BUCK_MODULE (Autodesk Fusion 360 design; units mm, degrees)
Autodesk Fusion 360 part; units mm, degrees
note: some values were not read from the file. Set by a fixed rule: which sketch regions a step uses.
sketch "Esquisse1" plane through (0, 0, 0) normal (0, 0, 1) x (1, 0, 0)
  line L0 (38, -53) -> (-38, -53)
  line L1 (-38, -53) -> (-38, 53)
  line L2 (-38, 53) -> (38, 53)
  line L3 (38, 53) -> (38, -53)
  line L4 (38, -53) -> (-38, 53) construction
  line L5 (-38, -53) -> (38, 53) construction
  dimension "d1" = 76
  dimension "d2" = 106
  constraint horizontal L0
  constraint perpendicular L0 L1
  constraint parallel L0 L2
  constraint parallel L1 L3
  constraint coincident L4 origin
  constraint coincident L5 origin
  measures "d1" distance of L1.end L2.end
  measures "d2" distance of L0.end L1.end
extrude "Extrusion1" add sketch "Esquisse1" along normal blind 40
sketch "Esquisse2" plane through (0, 0, 0) normal (0, 0, -1) x (1, 0, 0)
  line L0 (-38, -53) -> (38, -53)
  line L1 (38, -53) -> (38, 53)
  line L2 (38, 53) -> (-38, 53)
  line L3 (-38, 53) -> (-38, -53)
  line L4 (34.75, -38) -> (-34.75, -38)
  line L5 (-34.75, -38) -> (-34.75, 49)
  line L6 (-34.75, 49) -> (34.75, 49)
  line L7 (34.75, 49) -> (34.75, -38)
  line L8 (34.75, -38) -> (-34.75, 49) construction
  line L9 (-34.75, -38) -> (34.75, 49) construction
  line L10 (-34.75, -38) -> (34.75, -38)
  line L11 (34.75, -38) -> (34.75, -49)
  line L12 (34.75, -49) -> (-34.75, -49)
  line L13 (-34.75, -49) -> (-34.75, -38)
  circle A0 centre (-34.75, 49) radius 1.6
  circle A1 centre (34.75, 49) radius 1.6
  circle A2 centre (-34.75, -49) radius 1.6
  circle A3 centre (34.75, -38) radius 1.6
  point P0 (0, 5.5)
  dimension "d5" = 69.5
  dimension "d6" = 87
  dimension "d7" = 11
  dimension "d8" = 69.5
  dimension "d9" = 4
  dimension "d10" = 3.25
  dimension "d11" = 3.2
  dimension "d12" = 3.2
  dimension "d13" = 3.2
  dimension "d14" = 3.2
  constraint horizontal L4
  constraint perpendicular L4 L5
  constraint parallel L4 L6
  constraint parallel L5 L7
  constraint coincident L8 P0
  constraint coincident L9 P0
  constraint horizontal L10
  constraint vertical L11
  constraint horizontal L12
  constraint vertical L13
  constraint coincident L5.end L6.start
  constraint coincident L6.end L7.start
  constraint coincident L12.end L13.start
  constraint coincident L4.start L7.end
  measures "d5" distance of L5.end L6.end
  measures "d6" distance of L4.end L5.end
  measures "d7" distance of L4.end L12.end
  measures "d8" distance of L4.end L4.start
  measures "d9" distance of L2 L6
  measures "d10" distance of L1 L7
  measures "d11" diameter of A0
  measures "d12" diameter of A1
  measures "d13" diameter of A2
  measures "d14" diameter of A3
extrude "Extrusion2" cut sketch "Esquisse2" against normal blind 5 contours L4 L10 L11 A3 | L4 L7 L10 A3 | L7 L11 A3 | L6 L7 A1 | L6 L7 A1 | L5 L6 A0 | L5 L6 A0 | L12 L13 A2 | L12 L13 A2
equation "d7 = 98 mm - 87 mm"
equation "d8 = d5"
equation "d9 = ( ( 106 - 98 ) / 2 ) * 1 mm"
equation "d10 = ( ( 76 - 69.5 ) / 2 ) * 1 mm"
